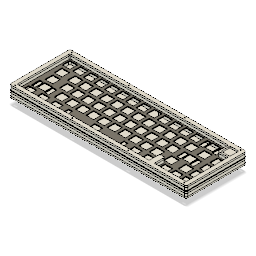
GoD68_Fusion360_Project (Autodesk Fusion 360 design; units mm, degrees)
Autodesk Fusion 360 part; units mm, degrees
(part 1 of 4)
sketch "草图1" plane through (0, 0, 0) normal (0, 1, 0) x (1, 0, 0)
  line L0 (318.896, 0.3693) -> (0.0951, 0.3693)
  line L1 (0.0951, 0.3693) -> (0.0951, 109.619)
  line L2 (0.0951, 109.619) -> (318.896, 109.619)
  line L3 (318.896, 109.619) -> (318.896, 0.3693)
sketch "草图2" plane through (0, 0, 125) normal (0, 1, 0) x (1, 0, 0)
  line L0 (154.495, 109.619) -> (154.495, 102.62)
  line L1 (164.495, 109.619) -> (318.896, 109.619)
  line L2 (311.895, 102.62) -> (164.495, 102.62)
  line L3 (318.896, 109.619) -> (318.896, 0.3693)
  line L4 (7.0941, 7.3697) -> (311.895, 7.3697)
  line L5 (0.0951, 0.3693) -> (0.0951, 109.619)
  line L6 (154.495, 102.62) -> (7.0942, 102.62)
  line L7 (7.0941, 102.62) -> (7.0941, 7.3697)
  line L8 (318.896, 0.3693) -> (0.0951, 0.3693)
  line L9 (311.895, 7.3697) -> (311.895, 102.62)
  line L10 (0.0951, 109.619) -> (154.495, 109.619)
  line L11 (164.495, 102.62) -> (164.495, 109.619)
sketch "草图3" plane through (0, 0, 250) normal (0, 1, 0) x (1, 0, 0)
  line L0 (264.413, 52.6948) -> (264.413, 47.9944)
  line L1 (278.412, 47.9944) -> (278.412, 52.6948)
  line L2 (279.937, 52.6948) -> (279.937, 48.2244)
  line L3 (262.887, 52.6948) -> (264.413, 52.6948)
  line L4 (52.4813, 42.9436) -> (66.482, 42.9436)
  line L5 (204.881, 28.9443) -> (204.881, 42.9436)
  line L6 (281.663, 48.2244) -> (281.663, 47.0242)
  line L7 (281.663, 47.0242) -> (284.963, 47.0242)
  line L8 (255.312, 54.4946) -> (256.137, 54.4946)
  line L9 (284.963, 47.0242) -> (284.963, 48.2244)
  line L10 (128.681, 28.9443) -> (128.681, 42.9436)
  line L11 (286.687, 48.2244) -> (286.687, 54.4946)
  line L12 (286.687, 54.4946) -> (287.512, 54.4946)
  line L13 (90.5813, 28.9443) -> (90.5813, 42.9436)
  line L14 (278.412, 52.6948) -> (279.937, 52.6948)
  line L15 (66.482, 28.9443) -> (52.4813, 28.9443)
  line L16 (256.137, 48.2244) -> (257.863, 48.2244)
  line L17 (71.5313, 42.9436) -> (85.532, 42.9436)
  line L18 (264.413, 47.9944) -> (278.412, 47.9944)
  line L19 (284.963, 48.2244) -> (286.687, 48.2244)
  line L20 (279.937, 48.2244) -> (281.663, 48.2244)
  line L21 (166.781, 42.9436) -> (180.782, 42.9436)
  line L22 (142.682, 28.9443) -> (128.681, 28.9443)
  line L23 (257.863, 48.2244) -> (257.863, 47.0242)
  line L24 (256.137, 54.4946) -> (256.137, 48.2244)
  line L25 (261.163, 48.2244) -> (262.887, 48.2244)
  line L26 (185.831, 42.9436) -> (199.832, 42.9436)
  line L27 (262.887, 60.5247) -> (256.137, 60.5247)
  line L28 (262.887, 48.2244) -> (262.887, 52.6948)
  line L29 (166.781, 28.9443) -> (166.781, 42.9436)
  line L30 (71.5313, 28.9443) -> (71.5313, 42.9436)
  line L31 (287.512, 57.2946) -> (286.687, 57.2946)
  line L32 (176.306, 47.9944) -> (176.306, 61.9936)
  line L33 (218.882, 42.9436) -> (218.882, 28.9443)
  line L34 (138.206, 47.9944) -> (138.206, 61.9936)
  line L35 (30.7619, 61.9936) -> (30.7619, 47.9944)
  line L36 (147.731, 42.9436) -> (161.732, 42.9436)
  line L37 (81.0563, 61.9936) -> (95.057, 61.9936)
  line L38 (109.631, 42.9436) -> (123.632, 42.9436)
  line L39 (180.782, 28.9443) -> (166.781, 28.9443)
  line L40 (85.532, 42.9436) -> (85.532, 28.9443)
  line L41 (133.157, 47.9944) -> (119.156, 47.9944)
  line L42 (286.687, 60.5247) -> (279.937, 60.5247)
  line L43 (85.532, 28.9443) -> (71.5313, 28.9443)
  line L44 (279.937, 57.2946) -> (278.412, 57.2946)
  line L45 (190.307, 61.9936) -> (190.307, 47.9944)
  line L46 (142.682, 42.9436) -> (142.682, 28.9443)
  line L47 (309.37, 61.9936) -> (309.37, 47.9944)
  line L48 (195.356, 47.9944) -> (195.356, 61.9936)
  line L49 (287.512, 54.4946) -> (287.512, 57.2946)
  line L50 (109.631, 28.9443) -> (109.631, 42.9436)
  line L51 (123.632, 42.9436) -> (123.632, 28.9443)
  line L52 (104.582, 28.9443) -> (90.5813, 28.9443)
  line L53 (42.9563, 47.9944) -> (42.9563, 61.9936)
  line L54 (209.357, 61.9936) -> (209.357, 47.9944)
  line L55 (100.106, 61.9936) -> (114.107, 61.9936)
  line L56 (119.156, 47.9944) -> (119.156, 61.9936)
  line L57 (161.732, 28.9443) -> (147.731, 28.9443)
  line L58 (228.407, 61.9936) -> (228.407, 47.9944)
  line L59 (95.057, 61.9936) -> (95.057, 47.9944)
  line L60 (95.057, 47.9944) -> (81.0563, 47.9944)
  line L61 (114.107, 61.9936) -> (114.107, 47.9944)
  line L62 (76.007, 47.9944) -> (62.0063, 47.9944)
  line L63 (152.207, 47.9944) -> (138.206, 47.9944)
  line L64 (309.37, 47.9944) -> (295.37, 47.9944)
  line L65 (56.957, 47.9944) -> (42.9563, 47.9944)
  line L66 (56.957, 61.9936) -> (56.957, 47.9944)
  line L67 (114.107, 47.9944) -> (100.106, 47.9944)
  line L68 (16.7624, 61.9936) -> (30.7619, 61.9936)
  line L69 (247.457, 47.9944) -> (233.456, 47.9944)
  line L70 (76.007, 61.9936) -> (76.007, 47.9944)
  line L71 (176.306, 61.9936) -> (190.307, 61.9936)
  line L72 (157.256, 61.9936) -> (171.257, 61.9936)
  line L73 (42.9563, 61.9936) -> (56.957, 61.9936)
  line L74 (214.406, 61.9936) -> (228.407, 61.9936)
  line L75 (171.257, 47.9944) -> (157.256, 47.9944)
  line L76 (233.456, 47.9944) -> (233.456, 61.9936)
  line L77 (62.0063, 61.9936) -> (76.007, 61.9936)
  line L78 (62.0063, 47.9944) -> (62.0063, 61.9936)
  line L79 (279.937, 60.5247) -> (279.937, 57.2946)
  line L80 (233.456, 61.9936) -> (247.457, 61.9936)
  line L81 (171.257, 61.9936) -> (171.257, 47.9944)
  line L82 (278.412, 61.9936) -> (264.413, 61.9936)
  line L83 (228.407, 47.9944) -> (214.406, 47.9944)
  line L84 (30.7619, 47.9944) -> (16.7624, 47.9944)
  line L85 (16.7624, 47.9944) -> (16.7624, 61.9936)
  line L86 (247.457, 61.9936) -> (247.457, 47.9944)
  line L87 (286.687, 57.2946) -> (286.687, 60.5247)
  line L88 (100.106, 47.9944) -> (100.106, 61.9936)
  line L89 (81.0563, 47.9944) -> (81.0563, 61.9936)
  line L90 (190.307, 47.9944) -> (176.306, 47.9944)
  line L91 (152.207, 61.9936) -> (152.207, 47.9944)
  line L92 (166.495, 67.0444) -> (152.495, 67.0444)
  line L93 (152.495, 67.0444) -> (152.495, 81.0436)
  line L94 (185.545, 81.0436) -> (185.545, 67.0444)
  line L95 (223.645, 67.0444) -> (209.645, 67.0444)
  line L96 (138.206, 61.9936) -> (152.207, 61.9936)
  line L97 (128.395, 81.0436) -> (128.395, 67.0444)
  line L98 (95.3452, 81.0436) -> (109.345, 81.0436)
  line L99 (109.345, 67.0444) -> (95.3452, 67.0444)
  line L100 (152.495, 81.0436) -> (166.495, 81.0436)
  line L101 (76.2953, 81.0436) -> (90.2945, 81.0436)
  line L102 (157.256, 47.9944) -> (157.256, 61.9936)
  line L103 (223.645, 81.0436) -> (223.645, 67.0444)
  line L104 (278.412, 57.2946) -> (278.412, 61.9936)
  line L105 (133.157, 61.9936) -> (133.157, 47.9944)
  line L106 (295.37, 61.9936) -> (309.37, 61.9936)
  line L107 (119.156, 61.9936) -> (133.157, 61.9936)
  line L108 (14.3812, 81.0436) -> (28.3821, 81.0436)
  line L109 (242.695, 67.0444) -> (228.695, 67.0444)
  line L110 (295.37, 47.9944) -> (295.37, 61.9936)
  line L111 (309.37, 67.0444) -> (295.37, 67.0444)
  line L112 (271.556, 81.0436) -> (285.557, 81.0436)
  line L113 (209.357, 47.9944) -> (195.356, 47.9944)
  line L114 (171.545, 67.0444) -> (171.545, 81.0436)
  line L115 (228.695, 81.0436) -> (242.695, 81.0436)
  line L116 (195.356, 61.9936) -> (209.357, 61.9936)
  line L117 (309.37, 81.0436) -> (309.37, 67.0444)
  line L118 (295.37, 81.0436) -> (309.37, 81.0436)
  line L119 (214.406, 47.9944) -> (214.406, 61.9936)
  line L120 (295.37, 67.0444) -> (295.37, 81.0436)
  line L121 (114.395, 67.0444) -> (114.395, 81.0436)
  line L122 (95.3452, 67.0444) -> (95.3452, 81.0436)
  line L123 (228.695, 67.0444) -> (228.695, 81.0436)
  line L124 (38.1952, 67.0444) -> (38.1952, 81.0436)
  line L125 (242.695, 81.0436) -> (242.695, 67.0444)
  line L126 (52.1945, 67.0444) -> (38.1952, 67.0444)
  line L127 (247.745, 67.0444) -> (247.745, 81.0436)
  line L128 (109.345, 81.0436) -> (109.345, 67.0444)
  line L129 (265.269, 98.6247) -> (258.52, 98.6247)
  line L130 (258.52, 95.3961) -> (257.695, 95.3961)
  line L131 (57.2453, 67.0444) -> (57.2453, 81.0436)
  line L132 (285.557, 81.0436) -> (285.557, 67.0444)
  line L133 (266.795, 100.095) -> (266.795, 95.3961)
  line L134 (204.595, 67.0444) -> (190.595, 67.0444)
  line L135 (128.395, 67.0444) -> (114.395, 67.0444)
  line L136 (76.2953, 67.0444) -> (76.2953, 81.0436)
  line L137 (209.645, 81.0436) -> (223.645, 81.0436)
  line L138 (38.1952, 81.0436) -> (52.1945, 81.0436)
  line L139 (133.445, 67.0444) -> (133.445, 81.0436)
  line L140 (52.1945, 81.0436) -> (52.1945, 67.0444)
  line L141 (258.52, 98.6247) -> (258.52, 95.3961)
  line L142 (57.2453, 81.0436) -> (71.2445, 81.0436)
  line L143 (71.2445, 67.0444) -> (57.2453, 67.0444)
  line L144 (147.445, 81.0436) -> (147.445, 67.0444)
  line L145 (265.269, 95.3961) -> (265.269, 98.6247)
  line L146 (247.745, 81.0436) -> (261.745, 81.0436)
  line L147 (209.645, 67.0444) -> (209.645, 81.0436)
  line L148 (261.745, 81.0436) -> (261.745, 67.0444)
  line L149 (166.495, 81.0436) -> (166.495, 67.0444)
  line L150 (71.2445, 81.0436) -> (71.2445, 67.0444)
  line L151 (261.745, 67.0444) -> (247.745, 67.0444)
  line L152 (266.795, 86.0944) -> (280.795, 86.0944)
  line L153 (185.545, 67.0444) -> (171.545, 67.0444)
  line L154 (284.044, 86.3258) -> (284.044, 85.1256)
  line L155 (219.17, 100.095) -> (233.17, 100.095)
  line L156 (287.345, 86.3258) -> (289.07, 86.3258)
  line L157 (147.445, 67.0444) -> (133.445, 67.0444)
  line L158 (258.52, 92.5946) -> (258.52, 86.3258)
  line L159 (133.445, 81.0436) -> (147.445, 81.0436)
  line L160 (171.545, 81.0436) -> (185.545, 81.0436)
  line L161 (265.269, 86.3258) -> (265.269, 90.7948)
  line L162 (257.695, 95.3961) -> (257.695, 92.5946)
  line L163 (90.2945, 81.0436) -> (90.2945, 67.0444)
  line L164 (200.12, 86.0944) -> (200.12, 100.095)
  line L165 (204.595, 81.0436) -> (204.595, 67.0444)
  line L166 (123.919, 100.095) -> (137.92, 100.095)
  line L167 (287.345, 85.1256) -> (287.345, 86.3258)
  line L168 (289.07, 92.5946) -> (289.895, 92.5946)
  line L169 (280.795, 90.7948) -> (282.32, 90.7948)
  line L170 (190.595, 67.0444) -> (190.595, 81.0436)
  line L171 (90.2945, 67.0444) -> (76.2953, 67.0444)
  line L172 (257.695, 92.5946) -> (258.52, 92.5946)
  line L173 (14.3812, 67.0444) -> (14.3812, 81.0436)
  line L174 (266.795, 95.3961) -> (265.269, 95.3961)
  line L175 (28.3821, 67.0444) -> (14.3812, 67.0444)
  line L176 (271.556, 67.0444) -> (271.556, 81.0436)
  line L177 (114.395, 81.0436) -> (128.395, 81.0436)
  line L178 (252.22, 86.0944) -> (238.22, 86.0944)
  line L179 (28.3821, 81.0436) -> (28.3821, 67.0444)
  line L180 (285.557, 67.0444) -> (271.556, 67.0444)
  line L181 (190.595, 81.0436) -> (204.595, 81.0436)
  line L182 (219.17, 86.0944) -> (219.17, 100.095)
  line L183 (289.895, 92.5946) -> (289.895, 95.3961)
  line L184 (123.919, 86.0944) -> (123.919, 100.095)
  line L185 (280.795, 86.0944) -> (280.795, 90.7948)
  line L186 (233.17, 100.095) -> (233.17, 86.0944)
  line L187 (85.8203, 100.095) -> (99.8195, 100.095)
  line L188 (176.02, 100.095) -> (176.02, 86.0944)
  line L189 (142.97, 100.095) -> (156.97, 100.095)
  line L190 (156.97, 100.095) -> (156.97, 86.0944)
  line L191 (282.32, 98.6247) -> (282.32, 95.3961)
  line L192 (195.07, 86.0944) -> (181.07, 86.0944)
  line L193 (282.32, 95.3961) -> (280.795, 95.3961)
  line L194 (118.868, 86.0944) -> (104.869, 86.0944)
  line L195 (258.52, 86.3258) -> (260.244, 86.3258)
  line L196 (99.8195, 86.0944) -> (85.8203, 86.0944)
  line L197 (280.795, 95.3961) -> (280.795, 100.095)
  line L198 (156.97, 86.0944) -> (142.97, 86.0944)
  line L199 (118.868, 100.095) -> (118.868, 86.0944)
  line L200 (162.02, 86.0944) -> (162.02, 100.095)
  line L201 (289.07, 95.3961) -> (289.07, 98.6247)
  line L202 (263.544, 86.3258) -> (265.269, 86.3258)
  line L203 (195.07, 100.095) -> (195.07, 86.0944)
  line L204 (214.12, 86.0944) -> (200.12, 86.0944)
  line L205 (289.07, 98.6247) -> (282.32, 98.6247)
  line L206 (289.895, 95.3961) -> (289.07, 95.3961)
  line L207 (176.02, 86.0944) -> (162.02, 86.0944)
  line L208 (200.12, 100.095) -> (214.12, 100.095)
  line L209 (137.92, 86.0944) -> (123.919, 86.0944)
  line L210 (137.92, 100.095) -> (137.92, 86.0944)
  line L211 (233.17, 86.0944) -> (219.17, 86.0944)
  line L212 (260.244, 85.1256) -> (263.544, 85.1256)
  line L213 (47.7203, 86.0944) -> (47.7203, 100.095)
  line L214 (42.6695, 86.0944) -> (28.6701, 86.0944)
  line L215 (238.22, 100.095) -> (252.22, 100.095)
  line L216 (238.22, 86.0944) -> (238.22, 100.095)
  line L217 (289.07, 86.3258) -> (289.07, 92.5946)
  line L218 (142.97, 86.0944) -> (142.97, 100.095)
  line L219 (104.869, 86.0944) -> (104.869, 100.095)
  line L220 (284.044, 85.1256) -> (287.345, 85.1256)
  line L221 (99.8195, 100.095) -> (99.8195, 86.0944)
  line L222 (263.544, 85.1256) -> (263.544, 86.3258)
  line L223 (104.869, 100.095) -> (118.868, 100.095)
  line L224 (162.02, 100.095) -> (176.02, 100.095)
  line L225 (282.32, 90.7948) -> (282.32, 86.3258)
  line L226 (181.07, 100.095) -> (195.07, 100.095)
  line L227 (66.7703, 100.095) -> (80.7695, 100.095)
  line L228 (280.795, 100.095) -> (266.795, 100.095)
  line L229 (266.795, 90.7948) -> (266.795, 86.0944)
  line L230 (282.32, 86.3258) -> (284.044, 86.3258)
  line L231 (80.7695, 86.0944) -> (66.7703, 86.0944)
  line L232 (61.7195, 86.0944) -> (47.7203, 86.0944)
  line L233 (23.6196, 100.095) -> (23.6196, 86.0944)
  line L234 (9.6187, 86.0944) -> (9.6187, 100.095)
  line L235 (28.6701, 86.0944) -> (28.6701, 100.095)
  line L236 (265.269, 90.7948) -> (266.795, 90.7948)
  line L237 (85.8203, 86.0944) -> (85.8203, 100.095)
  line L238 (260.244, 86.3258) -> (260.244, 85.1256)
  line L239 (252.22, 100.095) -> (252.22, 86.0944)
  line L240 (214.12, 100.095) -> (214.12, 86.0944)
  line L241 (181.07, 86.0944) -> (181.07, 100.095)
  line L242 (47.7203, 100.095) -> (61.7195, 100.095)
  line L243 (42.6695, 100.095) -> (42.6695, 86.0944)
  line L244 (9.6187, 100.095) -> (23.6196, 100.095)
  line L245 (23.6196, 86.0944) -> (9.6187, 86.0944)
  line L246 (61.7195, 100.095) -> (61.7195, 86.0944)
  line L247 (66.7703, 86.0944) -> (66.7703, 100.095)
  line L248 (80.7695, 100.095) -> (80.7695, 86.0944)
  line L249 (28.6701, 100.095) -> (42.6695, 100.095)
  line L250 (191.437, 10.1258) -> (191.437, 16.3945)
  line L251 (271.27, 9.8943) -> (257.27, 9.8943)
  line L252 (131.063, 23.8938) -> (131.063, 19.1947)
  line L253 (145.062, 19.1947) -> (145.062, 23.8938)
  line L254 (186.413, 8.9242) -> (189.713, 8.9242)
  line L255 (145.062, 9.8943) -> (145.062, 14.5948)
  line L256 (295.37, 23.8938) -> (309.37, 23.8938)
  line L257 (91.4368, 22.4248) -> (84.6875, 22.4248)
  line L258 (189.713, 8.9242) -> (189.713, 10.1258)
  line L259 (131.063, 14.5948) -> (131.063, 9.8943)
  line L260 (86.4126, 10.1258) -> (86.4126, 8.9242)
  line L261 (184.687, 22.4248) -> (184.687, 19.1947)
  line L262 (84.6875, 16.3945) -> (84.6875, 10.1258)
  line L263 (145.062, 23.8938) -> (131.063, 23.8938)
  line L264 (295.37, 9.8943) -> (295.37, 23.8938)
  line L265 (83.862, 16.3945) -> (84.6875, 16.3945)
  line L266 (86.4126, 8.9242) -> (89.7132, 8.9242)
  line L267 (276.32, 23.8938) -> (290.32, 23.8938)
  line L268 (290.32, 23.8938) -> (290.32, 9.8943)
  line L269 (290.32, 9.8943) -> (276.32, 9.8943)
  line L270 (145.062, 14.5948) -> (184.687, 14.5948)
  line L271 (192.262, 16.3945) -> (192.262, 19.1947)
  line L272 (186.413, 10.1258) -> (186.413, 8.9242)
  line L273 (216.501, 9.8943) -> (202.5, 9.8943)
  line L274 (184.687, 19.1947) -> (145.062, 19.1947)
  line L275 (257.27, 9.8943) -> (257.27, 23.8938)
  line L276 (0.0951, 109.619) -> (318.896, 109.619)
  line L277 (240.312, 9.8943) -> (226.313, 9.8943)
  line L278 (226.313, 23.8938) -> (240.312, 23.8938)
  line L279 (91.4368, 10.1258) -> (91.4368, 14.5948)
  line L280 (202.5, 9.8943) -> (202.5, 23.8938)
  line L281 (59.6251, 23.8938) -> (73.6258, 23.8938)
  line L282 (191.437, 22.4248) -> (184.687, 22.4248)
  line L283 (309.37, 9.8943) -> (295.37, 9.8943)
  line L284 (84.6875, 10.1258) -> (86.4126, 10.1258)
  line L285 (83.862, 19.1947) -> (83.862, 16.3945)
  line L286 (309.37, 23.8938) -> (309.37, 9.8943)
  line L287 (191.437, 16.3945) -> (192.262, 16.3945)
  line L288 (184.687, 10.1258) -> (186.413, 10.1258)
  line L289 (184.687, 14.5948) -> (184.687, 10.1258)
  line L290 (192.262, 19.1947) -> (191.437, 19.1947)
  line L291 (226.313, 9.8943) -> (226.313, 23.8938)
  line L292 (202.5, 23.8938) -> (216.501, 23.8938)
  line L293 (0.0951, 0.3693) -> (0.0951, 109.619)
  line L294 (84.6875, 22.4248) -> (84.6875, 19.1947)
  line L295 (20.0008, 33.6448) -> (21.5249, 33.6448)
  line L296 (35.8126, 23.8938) -> (49.8119, 23.8938)
  line L297 (21.5249, 38.2446) -> (20.0008, 38.2446)
  line L298 (11.9999, 23.8938) -> (26.0008, 23.8938)
  line L299 (42.0758, 27.9742) -> (42.0758, 29.1744)
  line L300 (295.37, 28.9443) -> (295.37, 42.9436)
  line L301 (264.126, 28.9443) -> (250.125, 28.9443)
  line L302 (13.2498, 29.1744) -> (14.9751, 29.1744)
  line L303 (318.896, 109.619) -> (318.896, 0.3693)
  line L304 (290.32, 42.9436) -> (290.32, 28.9443)
  line L305 (264.126, 42.9436) -> (264.126, 28.9443)
  line L306 (91.4368, 19.1947) -> (91.4368, 22.4248)
  line L307 (43.8009, 35.4446) -> (44.625, 35.4446)
  line L308 (276.32, 28.9443) -> (276.32, 42.9436)
  line L309 (290.32, 28.9443) -> (276.32, 28.9443)
  line L310 (38.7752, 29.1744) -> (38.7752, 27.9742)
  line L311 (35.5258, 28.9443) -> (35.5258, 33.6448)
  line L312 (216.501, 23.8938) -> (216.501, 9.8943)
  line L313 (84.6875, 19.1947) -> (83.862, 19.1947)
  line L314 (250.125, 42.9436) -> (264.126, 42.9436)
  line L315 (189.713, 10.1258) -> (191.437, 10.1258)
  line L316 (37.0498, 41.4747) -> (37.0498, 38.2446)
  line L317 (257.27, 23.8938) -> (271.27, 23.8938)
  line L318 (91.4368, 14.5948) -> (131.063, 14.5948)
  line L319 (89.7132, 10.1258) -> (91.4368, 10.1258)
  line L320 (13.2498, 35.4446) -> (13.2498, 29.1744)
  line L321 (14.9751, 29.1744) -> (14.9751, 27.9742)
  line L322 (35.5258, 38.2446) -> (35.5258, 42.9436)
  line L323 (295.37, 42.9436) -> (309.37, 42.9436)
  line L324 (131.063, 19.1947) -> (91.4368, 19.1947)
  line L325 (26.0008, 23.8938) -> (26.0008, 9.8943)
  line L326 (18.2755, 29.1744) -> (20.0008, 29.1744)
  line L327 (318.896, 0.3693) -> (0.0951, 0.3693)
  line L328 (271.27, 23.8938) -> (271.27, 9.8943)
  line L329 (21.5249, 42.9436) -> (21.5249, 38.2446)
  line L330 (89.7132, 8.9242) -> (89.7132, 10.1258)
  line L331 (191.437, 19.1947) -> (191.437, 22.4248)
  line L332 (276.32, 42.9436) -> (290.32, 42.9436)
  line L333 (13.2498, 38.2446) -> (12.4258, 38.2446)
  line L334 (43.8009, 38.2446) -> (43.8009, 41.4747)
  line L335 (44.625, 35.4446) -> (44.625, 38.2446)
  line L336 (73.6258, 23.8938) -> (73.6258, 9.8943)
  line L337 (14.9751, 27.9742) -> (18.2755, 27.9742)
  line L338 (43.8009, 41.4747) -> (37.0498, 41.4747)
  line L339 (250.125, 28.9443) -> (250.125, 42.9436)
  line L340 (73.6258, 9.8943) -> (59.6251, 9.8943)
  line L341 (12.4258, 35.4446) -> (13.2498, 35.4446)
  line L342 (35.5258, 33.6448) -> (37.0498, 33.6448)
  line L343 (276.32, 9.8943) -> (276.32, 23.8938)
  line L344 (131.063, 9.8943) -> (145.062, 9.8943)
  line L345 (240.312, 23.8938) -> (240.312, 9.8943)
  line L346 (223.931, 42.9436) -> (237.932, 42.9436)
  line L347 (26.0008, 9.8943) -> (11.9999, 9.8943)
  line L348 (223.931, 28.9443) -> (223.931, 42.9436)
  line L349 (49.8119, 23.8938) -> (49.8119, 9.8943)
  line L350 (35.8126, 9.8943) -> (35.8126, 23.8938)
  line L351 (237.932, 28.9443) -> (223.931, 28.9443)
  line L352 (21.5249, 28.9443) -> (35.5258, 28.9443)
  line L353 (37.0498, 38.2446) -> (35.5258, 38.2446)
  line L354 (18.2755, 27.9742) -> (18.2755, 29.1744)
  line L355 (20.0008, 38.2446) -> (20.0008, 41.4747)
  line L356 (37.0498, 29.1744) -> (38.7752, 29.1744)
  line L357 (237.932, 42.9436) -> (237.932, 28.9443)
  line L358 (204.881, 42.9436) -> (218.882, 42.9436)
  line L359 (44.625, 38.2446) -> (43.8009, 38.2446)
  line L360 (43.8009, 29.1744) -> (43.8009, 35.4446)
  line L361 (38.7752, 27.9742) -> (42.0758, 27.9742)
  line L362 (20.0008, 29.1744) -> (20.0008, 33.6448)
  line L363 (49.8119, 9.8943) -> (35.8126, 9.8943)
  line L364 (11.9999, 9.8943) -> (11.9999, 23.8938)
  line L365 (42.0758, 29.1744) -> (43.8009, 29.1744)
  line L366 (309.37, 28.9443) -> (295.37, 28.9443)
  line L367 (59.6251, 9.8943) -> (59.6251, 23.8938)
  line L368 (20.0008, 41.4747) -> (13.2498, 41.4747)
  line L369 (13.2498, 41.4747) -> (13.2498, 38.2446)
  line L370 (35.5258, 42.9436) -> (21.5249, 42.9436)
  line L371 (309.37, 42.9436) -> (309.37, 28.9443)
  line L372 (37.0498, 33.6448) -> (37.0498, 29.1744)
  line L373 (12.4258, 38.2446) -> (12.4258, 35.4446)
  line L374 (185.831, 28.9443) -> (185.831, 42.9436)
  line L375 (123.632, 28.9443) -> (109.631, 28.9443)
  line L376 (218.882, 28.9443) -> (204.881, 28.9443)
  line L377 (90.5813, 42.9436) -> (104.582, 42.9436)
  line L378 (262.887, 57.2946) -> (262.887, 60.5247)
  line L379 (66.482, 42.9436) -> (66.482, 28.9443)
  line L380 (256.137, 60.5247) -> (256.137, 57.2946)
  line L381 (255.312, 57.2946) -> (255.312, 54.4946)
  line L382 (264.413, 61.9936) -> (264.413, 57.2946)
  line L383 (128.681, 42.9436) -> (142.682, 42.9436)
  line L384 (199.832, 28.9443) -> (185.831, 28.9443)
  line L385 (104.582, 42.9436) -> (104.582, 28.9443)
  line L386 (257.863, 47.0242) -> (261.163, 47.0242)
  line L387 (52.4813, 28.9443) -> (52.4813, 42.9436)
  line L388 (180.782, 42.9436) -> (180.782, 28.9443)
  line L389 (161.732, 42.9436) -> (161.732, 28.9443)
  line L390 (21.5249, 33.6448) -> (21.5249, 28.9443)
  line L391 (261.163, 47.0242) -> (261.163, 48.2244)
  line L392 (199.832, 42.9436) -> (199.832, 28.9443)
  line L393 (147.731, 28.9443) -> (147.731, 42.9436)
  line L394 (264.413, 57.2946) -> (262.887, 57.2946)
  line L395 (256.137, 57.2946) -> (255.312, 57.2946)
sketch "草图4" plane through (0, 0, 375) normal (0, 1, 0) x (1, 0, 0)
  line L0 (311.895, 102.62) -> (311.895, 7.3697)
  line L1 (0.0951, 0.3693) -> (0.0951, 109.619)
  line L2 (318.896, 109.619) -> (318.896, 0.3693)
  line L3 (311.895, 7.3697) -> (7.0942, 7.3697)
  line L4 (0.0951, 109.619) -> (318.896, 109.619)
  line L5 (7.0941, 7.3697) -> (7.0941, 102.62)
  line L6 (318.896, 0.3693) -> (0.0951, 0.3693)
  line L7 (7.0941, 102.62) -> (311.895, 102.62)
sketch "草图5" plane through (0, 0, 500) normal (0, 1, 0) x (1, 0, 0)
  line L0 (254.744, 7.3697) -> (311.895, 7.3697)
  line L1 (7.0928, 45.4685) -> (7.0942, 45.4685)
  line L2 (0.0951, 109.619) -> (318.896, 109.619)
  line L3 (311.895, 7.3697) -> (311.895, 83.5699)
  line L4 (7.0941, 64.5199) -> (7.0928, 64.5199)
  line L5 (7.0941, 7.3697) -> (245.22, 7.3697)
  line L6 (318.896, 0.3693) -> (0.0951, 0.3693)
  line L7 (7.0928, 64.5199) -> (7.0928, 45.4685)
  line L8 (7.0941, 83.5685) -> (7.0941, 64.5199)
  line L9 (292.845, 102.621) -> (7.0928, 102.621)
  line L10 (245.22, 26.4184) -> (254.744, 26.4184)
  line L11 (7.0928, 83.5685) -> (7.0942, 83.5685)
  line L12 (245.22, 7.3697) -> (245.22, 26.4184)
  line L13 (254.744, 26.4184) -> (254.744, 7.3697)
  line L14 (7.0941, 45.4685) -> (7.0941, 7.3697)
  line L15 (7.0928, 102.621) -> (7.0928, 83.5685)
  line L16 (292.845, 83.5699) -> (292.845, 102.621)
  line L17 (311.895, 83.5699) -> (292.845, 83.5699)
  line L18 (318.896, 109.619) -> (318.896, 0.3693)
  line L19 (0.0951, 0.3693) -> (0.0951, 109.619)
  line L20 (292.845, 102.621) -> (318.896, 102.621)
  line L21 (311.895, 83.5699) -> (311.895, 102.621)
  line L22 (245.22, 7.3697) -> (254.744, 7.3697)
  constraint coincident L18 L20.end
  constraint perpendicular L18 L20
  constraint coincident L20 L21.end
  constraint perpendicular L20 L21
  constraint perpendicular L12 L22
sketch "草图25" plane through (-325, 0, 150) normal (0, 1, 0) x (1, 0, 0)
  arc A0 (66.0312, -92.725) -> (66.5312, -92.225) centre (66.0312, -92.225) ccw
  line L0 (195.9063, -78.725) -> (208.9062, -78.725)
  arc A1 (84.4688, -80.225) -> (83.9688, -79.725) centre (83.9688, -80.225) ccw
  line L1 (250.675, -78.725) -> (263.675, -78.725)
  line L2 (124.4688, -78.725) -> (137.4688, -78.725)
  line L3 (177.9688, -79.725) -> (183.9688, -79.725)
  line L4 (77.4688, -80.225) -> (77.4688, -94.225)
  line L5 (184.4688, -80.225) -> (184.4688, -94.225)
  arc A2 (250.175, -92.225) -> (250.675, -92.725) centre (250.675, -92.225) ccw
  arc A3 (77.4688, -94.225) -> (77.9688, -94.725) centre (77.9688, -94.225) ccw
  arc A4 (124.4688, -78.725) -> (123.9688, -79.225) centre (124.4688, -79.225) ccw
  line L6 (195.9063, -92.725) -> (208.9062, -92.725)
  line L7 (77.9688, -94.725) -> (83.9688, -94.725)
  arc A5 (123.9688, -92.225) -> (124.4688, -92.725) centre (124.4688, -92.225) ccw
  line L8 (250.175, -79.225) -> (250.175, -92.225)
  arc A6 (219.2188, -92.225) -> (219.7188, -92.725) centre (219.7188, -92.225) ccw
  line L9 (209.4062, -79.225) -> (209.4062, -92.225)
  arc A7 (264.175, -79.225) -> (263.675, -78.725) centre (263.675, -79.225) ccw
  arc A8 (233.2188, -79.225) -> (232.7188, -78.725) centre (232.7188, -79.225) ccw
  arc A9 (83.9688, -94.725) -> (84.4688, -94.225) centre (83.9688, -94.225) ccw
  line L10 (250.675, -92.725) -> (263.675, -92.725)
  arc A10 (250.675, -78.725) -> (250.175, -79.225) centre (250.675, -79.225) ccw
  line L11 (124.4688, -92.725) -> (137.4688, -92.725)
  arc A11 (137.4688, -92.725) -> (137.9688, -92.225) centre (137.4688, -92.225) ccw
  arc A12 (184.4688, -80.225) -> (183.9688, -79.725) centre (183.9688, -80.225) ccw
  line L12 (84.4688, -80.225) -> (84.4688, -94.225)
  arc A13 (209.4062, -79.225) -> (208.9062, -78.725) centre (208.9062, -79.225) ccw
  arc A14 (219.7188, -78.725) -> (219.2188, -79.225) centre (219.7188, -79.225) ccw
  arc A15 (77.9688, -79.725) -> (77.4688, -80.225) centre (77.9688, -80.225) ccw
  line L13 (137.9688, -79.225) -> (137.9688, -92.225)
  line L14 (264.175, -79.225) -> (264.175, -92.225)
  arc A16 (183.9688, -94.725) -> (184.4688, -94.225) centre (183.9688, -94.225) ccw
  arc A17 (177.9688, -79.725) -> (177.4688, -80.225) centre (177.9688, -80.225) ccw
  line L15 (77.9688, -79.725) -> (83.9688, -79.725)
  arc A18 (195.9063, -78.725) -> (195.4063, -79.225) centre (195.9063, -79.225) ccw
  line L16 (177.4688, -80.225) -> (177.4688, -94.225)
  line L17 (123.9688, -79.225) -> (123.9688, -92.225)
  line L18 (177.9688, -94.725) -> (183.9688, -94.725)
  arc A19 (177.4688, -94.225) -> (177.9688, -94.725) centre (177.9688, -94.225) ccw
  arc A20 (195.4063, -92.225) -> (195.9063, -92.725) centre (195.9063, -92.225) ccw
  arc A21 (208.9062, -92.725) -> (209.4062, -92.225) centre (208.9062, -92.225) ccw
  line L19 (219.7188, -92.725) -> (232.7188, -92.725)
  line L20 (219.7188, -78.725) -> (232.7188, -78.725)
  line L21 (195.4063, -79.225) -> (195.4063, -92.225)
  line L22 (219.2188, -79.225) -> (219.2188, -92.225)
  arc A22 (232.7188, -92.725) -> (233.2188, -92.225) centre (232.7188, -92.225) ccw
  arc A23 (137.9688, -79.225) -> (137.4688, -78.725) centre (137.4688, -79.225) ccw
  arc A24 (269.725, -78.725) -> (269.225, -79.225) centre (269.725, -79.225) ccw
  line L23 (288.275, -79.225) -> (288.275, -92.225)
  line L24 (233.2188, -79.225) -> (233.2188, -92.225)
  line L25 (302.275, -79.225) -> (302.275, -92.225)
  arc A25 (302.275, -79.225) -> (301.775, -78.725) centre (301.775, -79.225) ccw
  line L26 (269.225, -79.225) -> (269.225, -92.225)
  line L27 (288.775, -92.725) -> (301.775, -92.725)
  arc A26 (282.725, -92.725) -> (283.225, -92.225) centre (282.725, -92.225) ccw
  arc A27 (269.225, -92.225) -> (269.725, -92.725) centre (269.725, -92.225) ccw
  arc A28 (288.775, -78.725) -> (288.275, -79.225) centre (288.775, -79.225) ccw
  line L28 (0, 0) -> (0, -95.25)
  line L29 (269.725, -92.725) -> (282.725, -92.725)
  line L30 (269.725, -78.725) -> (282.725, -78.725)
  line L31 (0, -95.25) -> (304.8, -95.25)
  arc A29 (283.225, -79.225) -> (282.725, -78.725) centre (282.725, -79.225) ccw
  arc A30 (301.775, -92.725) -> (302.275, -92.225) centre (301.775, -92.225) ccw
  line L32 (0, 0) -> (304.8, 0)
  arc A31 (263.675, -92.725) -> (264.175, -92.225) centre (263.675, -92.225) ccw
  line L33 (283.225, -79.225) -> (283.225, -92.225)
  line L34 (288.775, -78.725) -> (301.775, -78.725)
  arc A32 (288.275, -92.225) -> (288.775, -92.725) centre (288.775, -92.225) ccw
  arc A33 (83.9875, -59.675) -> (83.4875, -60.175) centre (83.9875, -60.175) ccw
  line L35 (304.8, 0) -> (304.8, -95.25)
  arc A34 (14.9313, -59.675) -> (14.4313, -60.175) centre (14.9313, -60.175) ccw
  arc A35 (27.9312, -73.675) -> (28.4312, -73.175) centre (27.9312, -73.175) ccw
  arc A36 (279.7568, -42.125) -> (279.2568, -41.625) centre (279.2568, -42.125) ccw
  arc A37 (272.7568, -56.125) -> (273.2568, -56.625) centre (273.2568, -56.125) ccw
  line L36 (14.9313, -73.675) -> (27.9312, -73.675)
  arc A38 (255.3808, -56.625) -> (255.8808, -56.125) centre (255.3808, -56.125) ccw
  arc A39 (288.275, -54.125) -> (288.775, -54.625) centre (288.775, -54.125) ccw
  line L37 (249.3808, -41.625) -> (255.3808, -41.625)
  arc A40 (5.9932, -75.175) -> (6.4933, -75.675) centre (6.4933, -75.175) ccw
  line L38 (288.275, -41.125) -> (288.275, -54.125)
  arc A41 (45.8875, -59.675) -> (45.3875, -60.175) centre (45.8875, -60.175) ccw
  line L39 (29.8693, -61.175) -> (29.8693, -75.175)
  arc A42 (45.3875, -73.175) -> (45.8875, -73.675) centre (45.8875, -73.175) ccw
  line L40 (12.9932, -61.175) -> (12.9932, -75.175)
  line L41 (14.9313, -59.675) -> (27.9312, -59.675)
  line L42 (249.3808, -56.625) -> (255.3808, -56.625)
  line L43 (59.3875, -60.175) -> (59.3875, -73.175)
  line L44 (64.9375, -59.675) -> (77.9375, -59.675)
  arc A43 (255.8808, -42.125) -> (255.3808, -41.625) centre (255.3808, -42.125) ccw
  line L45 (288.775, -40.625) -> (301.775, -40.625)
  line L46 (36.8693, -61.175) -> (36.8693, -75.175)
  arc A44 (14.4313, -73.175) -> (14.9313, -73.675) centre (14.9313, -73.175) ccw
  line L47 (14.4313, -60.175) -> (14.4313, -73.175)
  arc A45 (30.3693, -60.675) -> (29.8693, -61.175) centre (30.3693, -61.175) ccw
  line L48 (45.3875, -60.175) -> (45.3875, -73.175)
  line L49 (288.775, -54.625) -> (301.775, -54.625)
  arc A46 (29.8693, -75.175) -> (30.3693, -75.675) centre (30.3693, -75.175) ccw
  line L50 (45.8875, -73.675) -> (58.8875, -73.675)
  line L51 (30.3693, -60.675) -> (36.3693, -60.675)
  arc A47 (36.8693, -61.175) -> (36.3693, -60.675) centre (36.3693, -61.175) ccw
  arc A48 (6.4933, -60.675) -> (5.9933, -61.175) centre (6.4933, -61.175) ccw
  arc A49 (279.2568, -56.625) -> (279.7568, -56.125) centre (279.2568, -56.125) ccw
  arc A50 (248.8808, -56.125) -> (249.3808, -56.625) centre (249.3808, -56.125) ccw
  arc A51 (59.3875, -60.175) -> (58.8875, -59.675) centre (58.8875, -60.175) ccw
  arc A52 (78.4375, -60.175) -> (77.9375, -59.675) centre (77.9375, -60.175) ccw
  line L52 (64.4375, -60.175) -> (64.4375, -73.175)
  line L53 (28.4313, -60.175) -> (28.4312, -73.175)
  arc A53 (249.3808, -41.625) -> (248.8808, -42.125) centre (249.3808, -42.125) ccw
  arc A54 (64.4375, -73.175) -> (64.9375, -73.675) centre (64.9375, -73.175) ccw
  line L54 (248.8808, -42.125) -> (248.8808, -56.125)
  line L55 (64.9375, -73.675) -> (77.9375, -73.675)
  line L56 (83.9875, -59.675) -> (96.9875, -59.675)
  arc A55 (288.775, -40.625) -> (288.275, -41.125) centre (288.775, -41.125) ccw
  line L57 (6.4933, -60.675) -> (12.4932, -60.675)
  arc A56 (77.9375, -73.675) -> (78.4375, -73.175) centre (77.9375, -73.175) ccw
  line L58 (255.8808, -42.125) -> (255.8808, -56.125)
  arc A57 (58.8875, -73.675) -> (59.3875, -73.175) centre (58.8875, -73.175) ccw
  arc A58 (12.9932, -61.175) -> (12.4932, -60.675) centre (12.4932, -61.175) ccw
  arc A59 (302.275, -41.125) -> (301.775, -40.625) centre (301.775, -41.125) ccw
  line L59 (5.9932, -61.175) -> (5.9932, -75.175)
  line L60 (302.275, -41.125) -> (302.275, -54.125)
  arc A60 (64.9375, -59.675) -> (64.4375, -60.175) centre (64.9375, -60.175) ccw
  arc A61 (301.775, -54.625) -> (302.275, -54.125) centre (301.775, -54.125) ccw
  arc A62 (12.4932, -75.675) -> (12.9932, -75.175) centre (12.4932, -75.175) ccw
  arc A63 (36.3693, -75.675) -> (36.8693, -75.175) centre (36.3693, -75.175) ccw
  line L61 (30.3693, -75.675) -> (36.3693, -75.675)
  arc A64 (121.5875, -73.175) -> (122.0875, -73.675) centre (122.0875, -73.175) ccw
  line L62 (160.1875, -73.675) -> (173.1875, -73.675)
  line L63 (83.4875, -60.175) -> (83.4875, -73.175)
  line L64 (78.4375, -60.175) -> (78.4375, -73.175)
  line L65 (141.1375, -59.675) -> (154.1375, -59.675)
  line L66 (197.7875, -60.175) -> (197.7875, -73.175)
  line L67 (216.8375, -60.175) -> (216.8375, -73.175)
  line L68 (198.2875, -59.675) -> (211.2875, -59.675)
  line L69 (6.4933, -75.675) -> (12.4932, -75.675)
  arc A65 (173.6875, -60.175) -> (173.1875, -59.675) centre (173.1875, -60.175) ccw
  arc A66 (173.1875, -73.675) -> (173.6875, -73.175) centre (173.1875, -73.175) ccw
  line L70 (198.2875, -73.675) -> (211.2875, -73.675)
  line L71 (159.6875, -60.175) -> (159.6875, -73.175)
  line L72 (45.8875, -59.675) -> (58.8875, -59.675)
  arc A67 (230.3375, -73.675) -> (230.8375, -73.175) centre (230.3375, -73.175) ccw
  line L73 (102.5375, -60.175) -> (102.5375, -73.175)
  line L74 (217.3375, -73.675) -> (230.3375, -73.675)
  arc A68 (141.1375, -59.675) -> (140.6375, -60.175) centre (141.1375, -60.175) ccw
  arc A69 (135.5875, -60.175) -> (135.0875, -59.675) centre (135.0875, -60.175) ccw
  arc A70 (243.5313, -59.675) -> (243.0313, -60.175) centre (243.5313, -60.175) ccw
  line L75 (103.0375, -73.675) -> (116.0375, -73.675)
  arc A71 (97.4875, -60.175) -> (96.9875, -59.675) centre (96.9875, -60.175) ccw
  arc A72 (28.4312, -60.175) -> (27.9312, -59.675) centre (27.9312, -60.175) ccw
  line L76 (192.7375, -60.175) -> (192.7375, -73.175)
  arc A73 (198.2875, -59.675) -> (197.7875, -60.175) centre (198.2875, -60.175) ccw
  line L77 (243.5313, -73.675) -> (256.5313, -73.675)
  arc A74 (159.6875, -73.175) -> (160.1875, -73.675) centre (160.1875, -73.175) ccw
  arc A75 (154.6375, -60.175) -> (154.1375, -59.675) centre (154.1375, -60.175) ccw
  line L78 (173.6875, -60.175) -> (173.6875, -73.175)
  line L79 (83.9875, -73.675) -> (96.9875, -73.675)
  line L80 (217.3375, -59.675) -> (230.3375, -59.675)
  line L81 (97.4875, -60.175) -> (97.4875, -73.175)
  arc A76 (116.5375, -60.175) -> (116.0375, -59.675) centre (116.0375, -60.175) ccw
  arc A77 (103.0375, -59.675) -> (102.5375, -60.175) centre (103.0375, -60.175) ccw
  line L82 (179.2375, -73.675) -> (192.2375, -73.675)
  line L83 (178.7375, -60.175) -> (178.7375, -73.175)
  arc A78 (122.0875, -59.675) -> (121.5875, -60.175) centre (122.0875, -60.175) ccw
  arc A79 (160.1875, -59.675) -> (159.6875, -60.175) centre (160.1875, -60.175) ccw
  arc A80 (192.7375, -60.175) -> (192.2375, -59.675) centre (192.2375, -60.175) ccw
  line L84 (141.1375, -73.675) -> (154.1375, -73.675)
  arc A81 (211.7875, -60.175) -> (211.2875, -59.675) centre (211.2875, -60.175) ccw
  arc A82 (96.9875, -73.675) -> (97.4875, -73.175) centre (96.9875, -73.175) ccw
  line L85 (179.2375, -59.675) -> (192.2375, -59.675)
  arc A83 (178.7375, -73.175) -> (179.2375, -73.675) centre (179.2375, -73.175) ccw
  arc A84 (179.2375, -59.675) -> (178.7375, -60.175) centre (179.2375, -60.175) ccw
  line L86 (211.7875, -60.175) -> (211.7875, -73.175)
  line L87 (230.8375, -60.175) -> (230.8375, -73.175)
  arc A85 (140.6375, -73.175) -> (141.1375, -73.675) centre (141.1375, -73.175) ccw
  arc A86 (135.0875, -73.675) -> (135.5875, -73.175) centre (135.0875, -73.175) ccw
  arc A87 (116.0375, -73.675) -> (116.5375, -73.175) centre (116.0375, -73.175) ccw
  line L88 (135.5875, -60.175) -> (135.5875, -73.175)
  line L89 (122.0875, -73.675) -> (135.0875, -73.675)
  arc A88 (269.725, -59.675) -> (269.225, -60.175) centre (269.725, -60.175) ccw
  arc A89 (283.225, -60.175) -> (282.725, -59.675) centre (282.725, -60.175) ccw
  line L90 (269.725, -73.675) -> (282.725, -73.675)
  arc A90 (269.225, -73.175) -> (269.725, -73.675) centre (269.725, -73.175) ccw
  line L91 (5.4062, -78.725) -> (18.4063, -78.725)
  line L92 (257.0312, -60.175) -> (257.0312, -73.175)
  line L93 (154.6375, -60.175) -> (154.6375, -73.175)
  arc A91 (288.775, -59.675) -> (288.275, -60.175) centre (288.775, -60.175) ccw
  line L94 (140.6375, -60.175) -> (140.6375, -73.175)
  line L95 (302.275, -60.175) -> (302.275, -73.175)
  line L96 (269.725, -59.675) -> (282.725, -59.675)
  arc A92 (302.275, -60.175) -> (301.775, -59.675) centre (301.775, -60.175) ccw
  arc A93 (288.275, -73.175) -> (288.775, -73.675) centre (288.775, -73.175) ccw
  arc A94 (282.725, -73.675) -> (283.225, -73.175) centre (282.725, -73.175) ccw
  arc A95 (301.775, -73.675) -> (302.275, -73.175) centre (301.775, -73.175) ccw
  line L97 (288.275, -60.175) -> (288.275, -73.175)
  line L98 (160.1875, -59.675) -> (173.1875, -59.675)
  line L99 (288.775, -59.675) -> (301.775, -59.675)
  line L100 (5.4062, -92.725) -> (18.4063, -92.725)
  line L101 (18.9062, -79.225) -> (18.9062, -92.225)
  arc A96 (18.9062, -79.225) -> (18.4062, -78.725) centre (18.4062, -79.225) ccw
  arc A97 (216.8375, -73.175) -> (217.3375, -73.675) centre (217.3375, -73.175) ccw
  line L102 (269.225, -60.175) -> (269.225, -73.175)
  line L103 (288.775, -73.675) -> (301.775, -73.675)
  line L104 (4.9062, -79.225) -> (4.9062, -92.225)
  arc A98 (5.4062, -78.725) -> (4.9063, -79.225) centre (5.4062, -79.225) ccw
  arc A99 (4.9062, -92.225) -> (5.4062, -92.725) centre (5.4062, -92.225) ccw
  line L105 (283.225, -60.175) -> (283.225, -73.175)
  arc A100 (256.5312, -73.675) -> (257.0312, -73.175) centre (256.5312, -73.175) ccw
  arc A101 (243.0313, -73.175) -> (243.5313, -73.675) centre (243.5313, -73.175) ccw
  arc A102 (18.4062, -92.725) -> (18.9063, -92.225) centre (18.4062, -92.225) ccw
  line L106 (121.5875, -60.175) -> (121.5875, -73.175)
  line L107 (103.0375, -59.675) -> (116.0375, -59.675)
  line L108 (29.2188, -92.725) -> (42.2188, -92.725)
  line L109 (28.7188, -79.225) -> (28.7188, -92.225)
  line L110 (42.7188, -79.225) -> (42.7188, -92.225)
  arc A103 (154.1375, -73.675) -> (154.6375, -73.175) centre (154.1375, -73.175) ccw
  arc A104 (83.4875, -73.175) -> (83.9875, -73.675) centre (83.9875, -73.175) ccw
  line L111 (29.2188, -78.725) -> (42.2188, -78.725)
  arc A105 (29.2188, -78.725) -> (28.7188, -79.225) centre (29.2188, -79.225) ccw
  arc A106 (217.3375, -59.675) -> (216.8375, -60.175) centre (217.3375, -60.175) ccw
  arc A107 (211.2875, -73.675) -> (211.7875, -73.175) centre (211.2875, -73.175) ccw
  line L112 (122.0875, -59.675) -> (135.0875, -59.675)
  arc A108 (230.8375, -60.175) -> (230.3375, -59.675) centre (230.3375, -60.175) ccw
  arc A109 (102.5375, -73.175) -> (103.0375, -73.675) centre (103.0375, -73.175) ccw
  arc A110 (197.7875, -73.175) -> (198.2875, -73.675) centre (198.2875, -73.175) ccw
  line L113 (243.5313, -59.675) -> (256.5313, -59.675)
  line L114 (243.0312, -60.175) -> (243.0312, -73.175)
  arc A111 (192.2375, -73.675) -> (192.7375, -73.175) centre (192.2375, -73.175) ccw
  arc A112 (257.0312, -60.175) -> (256.5312, -59.675) centre (256.5312, -60.175) ccw
  line L115 (116.5375, -60.175) -> (116.5375, -73.175)
  arc A113 (73.175, -16.525) -> (73.675, -16.025) centre (73.175, -16.025) ccw
  line L116 (3.025, -16.525) -> (16.025, -16.525)
  arc A114 (41.125, -2.525) -> (40.625, -3.025) centre (41.125, -3.025) ccw
  line L117 (22.075, -16.525) -> (35.075, -16.525)
  arc A115 (60.175, -2.525) -> (59.675, -3.025) centre (60.175, -3.025) ccw
  line L118 (2.525, -3.025) -> (2.525, -16.025)
  line L119 (40.625, -3.025) -> (40.625, -16.025)
  line L120 (3.025, -2.525) -> (16.025, -2.525)
  line L121 (231.125, -3.025) -> (231.125, -16.025)
  arc A116 (16.025, -16.525) -> (16.525, -16.025) centre (16.025, -16.025) ccw
  line L122 (136.375, -16.525) -> (149.375, -16.525)
  line L123 (60.175, -2.525) -> (73.175, -2.525)
  line L124 (193.525, -16.525) -> (206.525, -16.525)
  line L125 (53.0313, -92.725) -> (66.0312, -92.725)
  arc A117 (116.825, -16.025) -> (117.325, -16.525) centre (117.325, -16.025) ccw
  line L126 (54.625, -3.025) -> (54.625, -16.025)
  arc A118 (149.875, -3.025) -> (149.375, -2.525) centre (149.375, -3.025) ccw
  arc A119 (207.025, -3.025) -> (206.525, -2.525) centre (206.525, -3.025) ccw
  arc A120 (98.275, -2.525) -> (97.775, -3.025) centre (98.275, -3.025) ccw
  arc A121 (78.725, -16.025) -> (79.225, -16.525) centre (79.225, -16.025) ccw
  line L127 (22.075, -2.525) -> (35.075, -2.525)
  line L128 (92.725, -3.025) -> (92.725, -16.025)
  arc A122 (73.675, -3.025) -> (73.175, -2.525) centre (73.175, -3.025) ccw
  line L129 (155.425, -16.525) -> (168.425, -16.525)
  line L130 (66.5312, -79.225) -> (66.5312, -92.225)
  line L131 (79.225, -16.525) -> (92.225, -16.525)
  arc A123 (54.125, -16.525) -> (54.625, -16.025) centre (54.125, -16.025) ccw
  line L132 (59.675, -3.025) -> (59.675, -16.025)
  arc A124 (92.725, -3.025) -> (92.225, -2.525) centre (92.225, -3.025) ccw
  line L133 (41.125, -16.525) -> (54.125, -16.525)
  arc A125 (52.5313, -92.225) -> (53.0313, -92.725) centre (53.0313, -92.225) ccw
  line L134 (73.675, -3.025) -> (73.675, -16.025)
  line L135 (78.725, -3.025) -> (78.725, -16.025)
  line L136 (98.275, -2.525) -> (111.275, -2.525)
  line L137 (41.125, -2.525) -> (54.125, -2.525)
  arc A126 (54.625, -3.025) -> (54.125, -2.525) centre (54.125, -3.025) ccw
  arc A127 (92.225, -16.525) -> (92.725, -16.025) centre (92.225, -16.025) ccw
  arc A128 (35.075, -16.525) -> (35.575, -16.025) centre (35.075, -16.025) ccw
  arc A129 (35.575, -3.025) -> (35.075, -2.525) centre (35.075, -3.025) ccw
  line L138 (187.975, -3.025) -> (187.975, -16.025)
  line L139 (52.5313, -79.225) -> (52.5313, -92.225)
  line L140 (16.525, -3.025) -> (16.525, -16.025)
  arc A130 (16.525, -3.025) -> (16.025, -2.525) centre (16.025, -3.025) ccw
  arc A131 (21.575, -16.025) -> (22.075, -16.525) centre (22.075, -16.025) ccw
  arc A132 (59.675, -16.025) -> (60.175, -16.525) centre (60.175, -16.025) ccw
  arc A133 (79.225, -2.525) -> (78.725, -3.025) centre (79.225, -3.025) ccw
  line L141 (79.225, -2.525) -> (92.225, -2.525)
  arc A134 (2.525, -16.025) -> (3.025, -16.525) centre (3.025, -16.025) ccw
  arc A135 (3.025, -2.525) -> (2.525, -3.025) centre (3.025, -3.025) ccw
  arc A136 (40.625, -16.025) -> (41.125, -16.525) centre (41.125, -16.025) ccw
  arc A137 (173.975, -16.025) -> (174.475, -16.525) centre (174.475, -16.025) ccw
  arc A138 (42.2188, -92.725) -> (42.7188, -92.225) centre (42.2188, -92.225) ccw
  arc A139 (193.525, -2.525) -> (193.025, -3.025) centre (193.525, -3.025) ccw
  line L142 (193.025, -3.025) -> (193.025, -16.025)
  arc A140 (22.075, -2.525) -> (21.575, -3.025) centre (22.075, -3.025) ccw
  arc A141 (28.7188, -92.225) -> (29.2188, -92.725) centre (29.2188, -92.225) ccw
  line L143 (53.0313, -78.725) -> (66.0312, -78.725)
  arc A142 (53.0313, -78.725) -> (52.5313, -79.225) centre (53.0313, -79.225) ccw
  arc A143 (66.5312, -79.225) -> (66.0312, -78.725) centre (66.0312, -79.225) ccw
  line L144 (60.175, -16.525) -> (73.175, -16.525)
  line L145 (21.575, -3.025) -> (21.575, -16.025)
  line L146 (35.575, -3.025) -> (35.575, -16.025)
  line L147 (98.275, -16.525) -> (111.275, -16.525)
  arc A144 (42.7188, -79.225) -> (42.2188, -78.725) centre (42.2188, -79.225) ccw
  arc A145 (130.825, -3.025) -> (130.325, -2.525) centre (130.325, -3.025) ccw
  line L148 (231.625, -16.525) -> (244.625, -16.525)
  line L149 (154.925, -3.025) -> (154.925, -16.025)
  arc A146 (117.325, -2.525) -> (116.825, -3.025) centre (117.325, -3.025) ccw
  line L150 (155.425, -2.525) -> (168.425, -2.525)
  line L151 (212.575, -2.525) -> (225.575, -2.525)
  line L152 (116.825, -3.025) -> (116.825, -16.025)
  arc A147 (174.475, -2.525) -> (173.975, -3.025) centre (174.475, -3.025) ccw
  arc A148 (149.375, -16.525) -> (149.875, -16.025) centre (149.375, -16.025) ccw
  line L153 (168.925, -3.025) -> (168.925, -16.025)
  line L154 (111.775, -3.025) -> (111.775, -16.025)
  arc A149 (97.775, -16.025) -> (98.275, -16.525) centre (98.275, -16.025) ccw
  line L155 (117.325, -16.525) -> (130.325, -16.525)
  arc A150 (231.125, -16.025) -> (231.625, -16.525) centre (231.625, -16.025) ccw
  line L156 (231.625, -2.525) -> (244.625, -2.525)
  arc A151 (187.975, -3.025) -> (187.475, -2.525) centre (187.475, -3.025) ccw
  arc A152 (212.575, -2.525) -> (212.075, -3.025) centre (212.575, -3.025) ccw
  line L157 (226.075, -3.025) -> (226.075, -16.025)
  arc A153 (244.625, -16.525) -> (245.125, -16.025) centre (244.625, -16.025) ccw
  line L158 (260.2, -16.525) -> (273.2, -16.525)
  arc A154 (187.475, -16.525) -> (187.975, -16.025) centre (187.475, -16.025) ccw
  line L159 (275.638, -3.525) -> (281.638, -3.525)
  line L160 (50.65, -21.575) -> (63.65, -21.575)
  arc A155 (102.25, -22.075) -> (101.75, -21.575) centre (101.75, -22.075) ccw
  line L161 (135.875, -3.025) -> (135.875, -16.025)
  arc A156 (212.075, -16.025) -> (212.575, -16.525) centre (212.575, -16.025) ccw
  line L162 (212.575, -16.525) -> (225.575, -16.525)
  arc A157 (245.125, -3.025) -> (244.625, -2.525) centre (244.625, -3.025) ccw
  line L163 (251.762, -18.525) -> (257.762, -18.525)
  arc A158 (226.075, -3.025) -> (225.575, -2.525) centre (225.575, -3.025) ccw
  line L164 (174.475, -16.525) -> (187.475, -16.525)
  arc A159 (111.775, -3.025) -> (111.275, -2.525) centre (111.275, -3.025) ccw
  arc A160 (135.875, -16.025) -> (136.375, -16.525) centre (136.375, -16.025) ccw
  line L165 (212.075, -3.025) -> (212.075, -16.025)
  line L166 (88.75, -35.575) -> (101.75, -35.575)
  arc A161 (282.138, -4.025) -> (281.638, -3.525) centre (281.638, -4.025) ccw
  line L167 (130.825, -3.025) -> (130.825, -16.025)
  line L168 (174.475, -2.525) -> (187.475, -2.525)
  line L169 (117.325, -2.525) -> (130.325, -2.525)
  arc A162 (155.425, -2.525) -> (154.925, -3.025) centre (155.425, -3.025) ccw
  line L170 (260.2, -2.525) -> (273.2, -2.525)
  line L171 (83.2, -22.075) -> (83.2, -35.075)
  arc A163 (21.2875, -22.075) -> (20.7875, -21.575) centre (20.7875, -22.075) ccw
  arc A164 (31.1, -35.075) -> (31.6, -35.575) centre (31.6, -35.075) ccw
  arc A165 (88.75, -21.575) -> (88.25, -22.075) centre (88.75, -22.075) ccw
  arc A166 (111.275, -16.525) -> (111.775, -16.025) centre (111.275, -16.025) ccw
  arc A167 (130.325, -16.525) -> (130.825, -16.025) centre (130.325, -16.025) ccw
  arc A168 (225.575, -16.525) -> (226.075, -16.025) centre (225.575, -16.025) ccw
  arc A169 (88.25, -35.075) -> (88.75, -35.575) centre (88.75, -35.075) ccw
  arc A170 (136.375, -2.525) -> (135.875, -3.025) centre (136.375, -3.025) ccw
  line L172 (193.525, -2.525) -> (206.525, -2.525)
  arc A171 (168.425, -16.525) -> (168.925, -16.025) centre (168.425, -16.025) ccw
  arc A172 (168.925, -3.025) -> (168.425, -2.525) centre (168.425, -3.025) ccw
  line L173 (149.875, -3.025) -> (149.875, -16.025)
  arc A173 (193.025, -16.025) -> (193.525, -16.525) centre (193.525, -16.025) ccw
  line L174 (97.775, -3.025) -> (97.775, -16.025)
  arc A174 (206.525, -16.525) -> (207.025, -16.025) centre (206.525, -16.025) ccw
  arc A175 (154.925, -16.025) -> (155.425, -16.525) centre (155.425, -16.025) ccw
  line L175 (245.125, -3.025) -> (245.125, -16.025)
  arc A176 (231.625, -2.525) -> (231.125, -3.025) centre (231.625, -3.025) ccw
  line L176 (136.375, -2.525) -> (149.375, -2.525)
  line L177 (207.025, -3.025) -> (207.025, -16.025)
  line L178 (173.975, -3.025) -> (173.975, -16.025)
  line L179 (50.65, -35.575) -> (63.65, -35.575)
  arc A177 (101.75, -35.575) -> (102.25, -35.075) centre (101.75, -35.075) ccw
  arc A178 (259.7, -16.025) -> (260.2, -16.525) centre (260.2, -16.025) ccw
  line L180 (258.262, -4.025) -> (258.262, -18.025)
  arc A179 (69.2, -35.075) -> (69.7, -35.575) centre (69.7, -35.075) ccw
  arc A180 (273.2, -16.525) -> (273.7, -16.025) centre (273.2, -16.025) ccw
  arc A181 (83.2, -22.075) -> (82.7, -21.575) centre (82.7, -22.075) ccw
  arc A182 (82.7, -35.575) -> (83.2, -35.075) centre (82.7, -35.075) ccw
  arc A183 (45.1, -22.075) -> (44.6, -21.575) centre (44.6, -22.075) ccw
  line L181 (88.75, -21.575) -> (101.75, -21.575)
  line L182 (31.6, -35.575) -> (44.6, -35.575)
  line L183 (31.1, -22.075) -> (31.1, -35.075)
  line L184 (69.2, -22.075) -> (69.2, -35.075)
  line L185 (88.25, -22.075) -> (88.25, -35.075)
  arc A184 (69.7, -21.575) -> (69.2, -22.075) centre (69.7, -22.075) ccw
  line L186 (45.1, -22.075) -> (45.1, -35.075)
  line L187 (140.35, -22.075) -> (140.35, -35.075)
  arc A185 (50.65, -21.575) -> (50.15, -22.075) centre (50.65, -22.075) ccw
  arc A186 (222.1, -21.575) -> (221.6, -22.075) centre (222.1, -22.075) ccw
  arc A187 (64.15, -22.075) -> (63.65, -21.575) centre (63.65, -22.075) ccw
  line L188 (107.8, -21.575) -> (120.8, -21.575)
  arc A188 (164.45, -35.075) -> (164.95, -35.575) centre (164.95, -35.075) ccw
  arc A189 (50.15, -35.075) -> (50.65, -35.575) centre (50.65, -35.075) ccw
  arc A190 (275.138, -18.025) -> (275.638, -18.525) centre (275.638, -18.025) ccw
  arc A191 (251.762, -3.525) -> (251.262, -4.025) centre (251.762, -4.025) ccw
  line L189 (273.7, -3.025) -> (273.7, -16.025)
  arc A192 (44.6, -35.575) -> (45.1, -35.075) centre (44.6, -35.075) ccw
  arc A193 (20.7875, -35.575) -> (21.2875, -35.075) centre (20.7875, -35.075) ccw
  line L190 (50.15, -22.075) -> (50.15, -35.075)
  line L191 (275.138, -4.025) -> (275.138, -18.025)
  arc A194 (126.35, -35.075) -> (126.85, -35.575) centre (126.85, -35.075) ccw
  arc A195 (197, -35.575) -> (197.5, -35.075) centre (197, -35.075) ccw
  line L192 (282.138, -4.025) -> (282.138, -18.025)
  line L193 (184, -21.575) -> (197, -21.575)
  line L194 (184, -35.575) -> (197, -35.575)
  line L195 (222.1, -35.575) -> (235.1, -35.575)
  line L196 (64.15, -22.075) -> (64.15, -35.075)
  line L197 (102.25, -22.075) -> (102.25, -35.075)
  line L198 (7.2875, -22.075) -> (7.2875, -35.075)
  line L199 (251.762, -3.525) -> (257.762, -3.525)
  line L200 (145.4, -22.075) -> (145.4, -35.075)